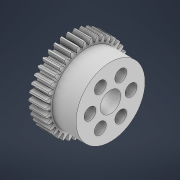
# Autodesk Inventor part: GearWheel
Saved by Autodesk Inventor 2022 (Build 260153000, 153)
## iProperties
Created: 2022-03-28
Part Number: GearWheel
Material: 一般
Document SubType Name: Modeling
Designer: neko2
Density: 1 g/cm^3
Appearance: 既定
Author: neko2
Autodesk Inventor part; units mm, degrees
(part 1 of 4)
ref_plane "YZ Plane" through (0, 0, 0) normal (1, 0, 0) x (0, 1, 0)
ref_plane "XZ Plane" through (0, 0, 0) normal (0, 1, 0) x (-1, 0, 0)
ref_plane "XY Plane" through (0, 0, 0) normal (0, 0, 1) x (1, 0, 0)
sketch "スケッチ1" plane through (0, 0, 0) normal (1, 0, 0) x (0, 1, 0)
  arc A0 (-4.4856, 2.8027) -> (-4.6292, 2.5586) centre (0, 0) ccw
  line L0 (-4.6292, 2.5586) -> (-4.6881, 2.5906)
  spline S0 degree 5 poles (-4.6881, 2.5906) (-4.6897, 2.5915) (-4.693, 2.5932) (-4.698, 2.5957) (-4.7047, 2.5989) (-4.7132, 2.6026) (-4.7219, 2.6061) (-4.7306, 2.6094) (-4.7393, 2.6127) (-4.7481, 2.6159) (-4.7569, 2.6191) (-4.7657, 2.6222) (-4.7746, 2.6252) (-4.7836, 2.6281) (-4.7926, 2.631) (-4.8016, 2.6337) (-4.8107, 2.6364) (-4.8198, 2.639) (-4.8289, 2.6415) (-4.8381, 2.644) (-4.8472, 2.6464) (-4.8565, 2.6488) (-4.8657, 2.6511) (-4.875, 2.6533) (-4.8843, 2.6555) (-4.8936, 2.6576) (-4.903, 2.6597) (-4.9124, 2.6617) (-4.9218, 2.6636) (-4.9313, 2.6656) (-4.9407, 2.6674) (-4.9502, 2.6692) (-4.9597, 2.671) (-4.9693, 2.6727) (-4.9788, 2.6743) (-4.9884, 2.6759) (-4.998, 2.6775) (-5.0076, 2.679) (-5.0173, 2.6804) (-5.027, 2.6818) (-5.0367, 2.6832) (-5.0464, 2.6845) (-5.0561, 2.6858) (-5.0658, 2.687) (-5.0756, 2.6882) (-5.0854, 2.6893) (-5.0952, 2.6904) (-5.105, 2.6915) (-5.1149, 2.6925) (-5.1248, 2.6934) (-5.1346, 2.6943) (-5.1445, 2.6952) (-5.1544, 2.696) (-5.1644, 2.6968) (-5.1743, 2.6976) (-5.1843, 2.6983) (-5.1943, 2.6989) (-5.2043, 2.6995) (-5.2143, 2.7001) (-5.2243, 2.7007) (-5.2344, 2.7012) (-5.2445, 2.7016) (-5.2545, 2.702) (-5.2646, 2.7024) (-5.2747, 2.7027) (-5.2849, 2.703) (-5.295, 2.7033) (-5.3052, 2.7035) (-5.3194, 2.7037) (-5.3316, 2.7039) (-5.3418, 2.704) (-5.35, 2.704) (-5.3562, 2.704) knots 0 0 0 0 0 0 0.014286 0.028571 0.042857 0.057143 0.071429 0.085714 0.1 0.114286 0.128571 0.142857 0.157143 0.171429 0.185714 0.2 0.214286 0.228571 0.242857 0.257143 0.271429 0.285714 0.3 0.314286 0.328571 0.342857 0.357143 0.371429 0.385714 0.4 0.414286 0.428571 0.442857 0.457143 0.471429 0.485714 0.5 0.514286 0.528571 0.542857 0.557143 0.571429 0.585714 0.6 0.614286 0.628571 0.642857 0.657143 0.671429 0.685714 0.7 0.714286 0.728571 0.742857 0.757143 0.771429 0.785714 0.8 0.814286 0.828571 0.842857 0.857143 0.871429 0.885714 0.9 0.914286 0.928571 0.942857 0.957143 1 1 1 1 1 1
  arc A1 (-5.3562, 2.704) -> (-5.4524, 2.5042) centre (0, 0) ccw
  spline S1 degree 5 poles (-4.9475, 2.0523) (-4.9492, 2.0531) (-4.9526, 2.0545) (-4.9576, 2.0569) (-4.9643, 2.0602) (-4.9725, 2.0645) (-4.9806, 2.0691) (-4.9886, 2.0738) (-4.9966, 2.0786) (-5.0046, 2.0835) (-5.0126, 2.0884) (-5.0206, 2.0934) (-5.0285, 2.0984) (-5.0363, 2.1036) (-5.0441, 2.1089) (-5.0519, 2.1142) (-5.0596, 2.1196) (-5.0673, 2.1252) (-5.075, 2.1307) (-5.0827, 2.1363) (-5.0903, 2.142) (-5.0979, 2.1478) (-5.1054, 2.1536) (-5.113, 2.1594) (-5.1205, 2.1653) (-5.128, 2.1713) (-5.1354, 2.1774) (-5.1428, 2.1835) (-5.1502, 2.1896) (-5.1576, 2.1958) (-5.165, 2.2021) (-5.1723, 2.2083) (-5.1796, 2.2147) (-5.1869, 2.2211) (-5.1941, 2.2275) (-5.2013, 2.234) (-5.2085, 2.2406) (-5.2157, 2.2472) (-5.2229, 2.2538) (-5.23, 2.2605) (-5.2371, 2.2672) (-5.2442, 2.274) (-5.2512, 2.2808) (-5.2583, 2.2877) (-5.2653, 2.2946) (-5.2723, 2.3016) (-5.2792, 2.3085) (-5.2862, 2.3156) (-5.2931, 2.3227) (-5.3, 2.3298) (-5.3068, 2.3369) (-5.3137, 2.3441) (-5.3205, 2.3514) (-5.3273, 2.3586) (-5.3341, 2.366) (-5.3409, 2.3733) (-5.3476, 2.3807) (-5.3543, 2.3882) (-5.361, 2.3956) (-5.3677, 2.4031) (-5.3743, 2.4107) (-5.381, 2.4183) (-5.3876, 2.4259) (-5.3942, 2.4336) (-5.4007, 2.4413) (-5.4073, 2.449) (-5.4138, 2.4568) (-5.4203, 2.4646) (-5.4294, 2.4756) (-5.4371, 2.4851) (-5.4435, 2.493) (-5.4486, 2.4994) (-5.4524, 2.5042) knots 0 0 0 0 0 0 0.014286 0.028571 0.042857 0.057143 0.071429 0.085714 0.1 0.114286 0.128571 0.142857 0.157143 0.171429 0.185714 0.2 0.214286 0.228571 0.242857 0.257143 0.271429 0.285714 0.3 0.314286 0.328571 0.342857 0.357143 0.371429 0.385714 0.4 0.414286 0.428571 0.442857 0.457143 0.471429 0.485714 0.5 0.514286 0.528571 0.542857 0.557143 0.571429 0.585714 0.6 0.614286 0.628571 0.642857 0.657143 0.671429 0.685714 0.7 0.714286 0.728571 0.742857 0.757143 0.771429 0.785714 0.8 0.814286 0.828571 0.842857 0.857143 0.871429 0.885714 0.9 0.914286 0.928571 0.942857 0.957143 1 1 1 1 1 1
  line L1 (-4.8857, 2.0262) -> (-4.9475, 2.0523)
  arc A2 (-4.8857, 2.0262) -> (-4.9872, 1.7617) centre (0, 0) ccw
  line L2 (-4.9872, 1.7617) -> (-5.0506, 1.7836)
  spline S2 degree 5 poles (-5.0506, 1.7836) (-5.0523, 1.7842) (-5.0558, 1.7854) (-5.0612, 1.7871) (-5.0683, 1.7891) (-5.0773, 1.7913) (-5.0864, 1.7933) (-5.0955, 1.7952) (-5.1047, 1.797) (-5.1139, 1.7987) (-5.1231, 1.8004) (-5.1323, 1.802) (-5.1416, 1.8035) (-5.1509, 1.805) (-5.1602, 1.8063) (-5.1696, 1.8075) (-5.179, 1.8086) (-5.1884, 1.8097) (-5.1978, 1.8107) (-5.2073, 1.8116) (-5.2167, 1.8125) (-5.2262, 1.8133) (-5.2357, 1.814) (-5.2452, 1.8147) (-5.2548, 1.8154) (-5.2643, 1.8159) (-5.2739, 1.8164) (-5.2835, 1.8168) (-5.2931, 1.8172) (-5.3027, 1.8175) (-5.3124, 1.8178) (-5.322, 1.818) (-5.3317, 1.8182) (-5.3414, 1.8183) (-5.3511, 1.8183) (-5.3608, 1.8183) (-5.3705, 1.8183) (-5.3803, 1.8182) (-5.39, 1.818) (-5.3998, 1.8178) (-5.4096, 1.8176) (-5.4194, 1.8173) (-5.4292, 1.8169) (-5.439, 1.8165) (-5.4489, 1.8161) (-5.4587, 1.8156) (-5.4685, 1.8151) (-5.4784, 1.8145) (-5.4883, 1.8138) (-5.4982, 1.8132) (-5.5081, 1.8124) (-5.518, 1.8117) (-5.5279, 1.8109) (-5.5378, 1.81) (-5.5478, 1.8091) (-5.5577, 1.8082) (-5.5677, 1.8072) (-5.5776, 1.8061) (-5.5876, 1.805) (-5.5976, 1.8039) (-5.6076, 1.8028) (-5.6176, 1.8016) (-5.6276, 1.8003) (-5.6376, 1.799) (-5.6477, 1.7977) (-5.6577, 1.7963) (-5.6677, 1.7949) (-5.6778, 1.7934) (-5.6919, 1.7913) (-5.704, 1.7895) (-5.714, 1.7878) (-5.7221, 1.7865) (-5.7282, 1.7855) knots 0 0 0 0 0 0 0.014286 0.028571 0.042857 0.057143 0.071429 0.085714 0.1 0.114286 0.128571 0.142857 0.157143 0.171429 0.185714 0.2 0.214286 0.228571 0.242857 0.257143 0.271429 0.285714 0.3 0.314286 0.328571 0.342857 0.357143 0.371429 0.385714 0.4 0.414286 0.428571 0.442857 0.457143 0.471429 0.485714 0.5 0.514286 0.528571 0.542857 0.557143 0.571429 0.585714 0.6 0.614286 0.628571 0.642857 0.657143 0.671429 0.685714 0.7 0.714286 0.728571 0.742857 0.757143 0.771429 0.785714 0.8 0.814286 0.828571 0.842857 0.857143 0.871429 0.885714 0.9 0.914286 0.928571 0.942857 0.957143 1 1 1 1 1 1
  arc A3 (-5.7282, 1.7855) -> (-5.7902, 1.5726) centre (0, 0) ccw
  spline S3 degree 5 poles (-5.2178, 1.21) (-5.2196, 1.2105) (-5.2232, 1.2114) (-5.2286, 1.2128) (-5.2357, 1.215) (-5.2445, 1.2179) (-5.2532, 1.2211) (-5.2619, 1.2244) (-5.2706, 1.2278) (-5.2793, 1.2313) (-5.288, 1.2348) (-5.2966, 1.2385) (-5.3053, 1.2422) (-5.3139, 1.246) (-5.3225, 1.2499) (-5.331, 1.2539) (-5.3395, 1.2579) (-5.348, 1.2621) (-5.3565, 1.2663) (-5.365, 1.2706) (-5.3734, 1.275) (-5.3819, 1.2794) (-5.3903, 1.2839) (-5.3987, 1.2884) (-5.4071, 1.293) (-5.4154, 1.2977) (-5.4238, 1.3024) (-5.4321, 1.3072) (-5.4404, 1.312) (-5.4487, 1.3169) (-5.457, 1.3219) (-5.4652, 1.3269) (-5.4735, 1.332) (-5.4817, 1.3371) (-5.4899, 1.3422) (-5.4981, 1.3475) (-5.5063, 1.3527) (-5.5144, 1.3581) (-5.5226, 1.3634) (-5.5307, 1.3689) (-5.5388, 1.3743) (-5.5469, 1.3798) (-5.555, 1.3854) (-5.5631, 1.391) (-5.5711, 1.3967) (-5.5792, 1.4024) (-5.5872, 1.4081) (-5.5952, 1.4139) (-5.6032, 1.4198) (-5.6112, 1.4256) (-5.6191, 1.4316) (-5.6271, 1.4376) (-5.635, 1.4436) (-5.6429, 1.4496) (-5.6508, 1.4557) (-5.6587, 1.4619) (-5.6665, 1.4681) (-5.6744, 1.4743) (-5.6822, 1.4806) (-5.69, 1.4869) (-5.6978, 1.4932) (-5.7056, 1.4996) (-5.7134, 1.5061) (-5.7212, 1.5125) (-5.7289, 1.519) (-5.7366, 1.5256) (-5.7443, 1.5322) (-5.752, 1.5388) (-5.7628, 1.5482) (-5.772, 1.5562) (-5.7796, 1.563) (-5.7857, 1.5685) (-5.7902, 1.5726) knots 0 0 0 0 0 0 0.014286 0.028571 0.042857 0.057143 0.071429 0.085714 0.1 0.114286 0.128571 0.142857 0.157143 0.171429 0.185714 0.2 0.214286 0.228571 0.242857 0.257143 0.271429 0.285714 0.3 0.314286 0.328571 0.342857 0.357143 0.371429 0.385714 0.4 0.414286 0.428571 0.442857 0.457143 0.471429 0.485714 0.5 0.514286 0.528571 0.542857 0.557143 0.571429 0.585714 0.6 0.614286 0.628571 0.642857 0.657143 0.671429 0.685714 0.7 0.714286 0.728571 0.742857 0.757143 0.771429 0.785714 0.8 0.814286 0.828571 0.842857 0.857143 0.871429 0.885714 0.9 0.914286 0.928571 0.942857 0.957143 1 1 1 1 1 1
  line L3 (-5.1526, 1.1944) -> (-5.2178, 1.21)
  arc A4 (-5.1526, 1.1944) -> (-5.2091, 0.9169) centre (0, 0) ccw
  line L4 (-5.2091, 0.9169) -> (-5.2752, 0.928)
  spline S4 degree 5 poles (-5.2752, 0.928) (-5.2771, 0.9283) (-5.2808, 0.9289) (-5.2863, 0.9296) (-5.2937, 0.9305) (-5.3029, 0.9312) (-5.3122, 0.9317) (-5.3215, 0.932) (-5.3308, 0.9323) (-5.3402, 0.9325) (-5.3496, 0.9326) (-5.3589, 0.9327) (-5.3683, 0.9327) (-5.3777, 0.9325) (-5.3872, 0.9323) (-5.3966, 0.9319) (-5.406, 0.9315) (-5.4155, 0.931) (-5.4249, 0.9304) (-5.4344, 0.9298) (-5.4439, 0.9291) (-5.4534, 0.9284) (-5.4629, 0.9275) (-5.4724, 0.9266) (-5.4819, 0.9257) (-5.4914, 0.9247) (-5.501, 0.9236) (-5.5105, 0.9224) (-5.52, 0.9212) (-5.5296, 0.9199) (-5.5391, 0.9186) (-5.5487, 0.9173) (-5.5583, 0.9158) (-5.5678, 0.9143) (-5.5774, 0.9128) (-5.587, 0.9112) (-5.5966, 0.9095) (-5.6062, 0.9078) (-5.6158, 0.9061) (-5.6254, 0.9043) (-5.635, 0.9024) (-5.6446, 0.9005) (-5.6542, 0.8985) (-5.6638, 0.8965) (-5.6735, 0.8945) (-5.6831, 0.8924) (-5.6927, 0.8902) (-5.7023, 0.888) (-5.712, 0.8858) (-5.7216, 0.8835) (-5.7313, 0.8811) (-5.7409, 0.8787) (-5.7506, 0.8763) (-5.7602, 0.8738) (-5.7699, 0.8713) (-5.7795, 0.8687) (-5.7892, 0.8661) (-5.7988, 0.8634) (-5.8085, 0.8607) (-5.8182, 0.858) (-5.8278, 0.8552) (-5.8375, 0.8524) (-5.8472, 0.8495) (-5.8568, 0.8466) (-5.8665, 0.8436) (-5.8762, 0.8406) (-5.8859, 0.8375) (-5.8955, 0.8344) (-5.9091, 0.83) (-5.9207, 0.8262) (-5.9304, 0.823) (-5.9381, 0.8203) (-5.9439, 0.8183) knots 0 0 0 0 0 0 0.014286 0.028571 0.042857 0.057143 0.071429 0.085714 0.1 0.114286 0.128571 0.142857 0.157143 0.171429 0.185714 0.2 0.214286 0.228571 0.242857 0.257143 0.271429 0.285714 0.3 0.314286 0.328571 0.342857 0.357143 0.371429 0.385714 0.4 0.414286 0.428571 0.442857 0.457143 0.471429 0.485714 0.5 0.514286 0.528571 0.542857 0.557143 0.571429 0.585714 0.6 0.614286 0.628571 0.642857 0.657143 0.671429 0.685714 0.7 0.714286 0.728571 0.742857 0.757143 0.771429 0.785714 0.8 0.814286 0.828571 0.842857 0.857143 0.871429 0.885714 0.9 0.914286 0.928571 0.942857 0.957143 1 1 1 1 1 1
  arc A5 (-5.9439, 0.8183) -> (-5.9701, 0.5981) centre (0, 0) ccw
  spline S5 degree 5 poles (-5.3458, 0.3347) (-5.3476, 0.3348) (-5.3513, 0.3351) (-5.3569, 0.3357) (-5.3643, 0.3366) (-5.3734, 0.3381) (-5.3826, 0.3398) (-5.3917, 0.3416) (-5.4008, 0.3436) (-5.41, 0.3456) (-5.4191, 0.3476) (-5.4282, 0.3498) (-5.4374, 0.352) (-5.4465, 0.3543) (-5.4556, 0.3568) (-5.4647, 0.3593) (-5.4737, 0.3619) (-5.4828, 0.3646) (-5.4919, 0.3674) (-5.5009, 0.3702) (-5.51, 0.3731) (-5.519, 0.3761) (-5.5281, 0.3791) (-5.5371, 0.3822) (-5.5461, 0.3854) (-5.5551, 0.3886) (-5.5642, 0.3919) (-5.5732, 0.3953) (-5.5822, 0.3987) (-5.5911, 0.4022) (-5.6001, 0.4057) (-5.6091, 0.4093) (-5.6181, 0.4129) (-5.627, 0.4166) (-5.636, 0.4203) (-5.6449, 0.4241) (-5.6538, 0.428) (-5.6628, 0.4319) (-5.6717, 0.4358) (-5.6806, 0.4399) (-5.6895, 0.4439) (-5.6984, 0.448) (-5.7073, 0.4522) (-5.7162, 0.4564) (-5.725, 0.4606) (-5.7339, 0.4649) (-5.7428, 0.4693) (-5.7516, 0.4737) (-5.7604, 0.4781) (-5.7693, 0.4826) (-5.7781, 0.4872) (-5.7869, 0.4918) (-5.7957, 0.4964) (-5.8045, 0.5011) (-5.8133, 0.5058) (-5.8221, 0.5106) (-5.8309, 0.5154) (-5.8397, 0.5202) (-5.8484, 0.5251) (-5.8572, 0.53) (-5.8659, 0.535) (-5.8746, 0.5401) (-5.8834, 0.5451) (-5.8921, 0.5502) (-5.9008, 0.5554) (-5.9095, 0.5606) (-5.9182, 0.5658) (-5.9269, 0.5711) (-5.939, 0.5785) (-5.9494, 0.585) (-5.958, 0.5904) (-5.9649, 0.5948) (-5.9701, 0.5981) knots 0 0 0 0 0 0 0.014286 0.028571 0.042857 0.057143 0.071429 0.085714 0.1 0.114286 0.128571 0.142857 0.157143 0.171429 0.185714 0.2 0.214286 0.228571 0.242857 0.257143 0.271429 0.285714 0.3 0.314286 0.328571 0.342857 0.357143 0.371429 0.385714 0.4 0.414286 0.428571 0.442857 0.457143 0.471429 0.485714 0.5 0.514286 0.528571 0.542857 0.557143 0.571429 0.585714 0.6 0.614286 0.628571 0.642857 0.657143 0.671429 0.685714 0.7 0.714286 0.728571 0.742857 0.757143 0.771429 0.785714 0.8 0.814286 0.828571 0.842857 0.857143 0.871429 0.885714 0.9 0.914286 0.928571 0.942857 0.957143 1 1 1 1 1 1
  line L5 (-5.2789, 0.33) -> (-5.3458, 0.3347)
  arc A6 (-5.2789, 0.33) -> (-5.289, 0.047) centre (0, 0) ccw
  line L6 (-5.289, 0.047) -> (-5.356, 0.0471)
  spline S6 degree 5 poles (-5.356, 0.0471) (-5.3579, 0.0471) (-5.3616, 0.047) (-5.3672, 0.0469) (-5.3746, 0.0465) (-5.3839, 0.0456) (-5.3931, 0.0446) (-5.4023, 0.0434) (-5.4116, 0.0421) (-5.4208, 0.0408) (-5.4301, 0.0394) (-5.4394, 0.0379) (-5.4486, 0.0363) (-5.4579, 0.0347) (-5.4671, 0.0329) (-5.4764, 0.031) (-5.4856, 0.029) (-5.4949, 0.027) (-5.5041, 0.0248) (-5.5133, 0.0227) (-5.5226, 0.0204) (-5.5318, 0.0181) (-5.541, 0.0157) (-5.5503, 0.0133) (-5.5595, 0.0108) (-5.5687, 0.0082) (-5.5779, 0.0055) (-5.5872, 0.0028) (-5.5964, 0.0001) (-5.6056, -0.0027) (-5.6148, -0.0056) (-5.624, -0.0085) (-5.6332, -0.0115) (-5.6424, -0.0146) (-5.6516, -0.0177) (-5.6608, -0.0208) (-5.67, -0.024) (-5.6791, -0.0273) (-5.6883, -0.0306) (-5.6975, -0.034) (-5.7067, -0.0374) (-5.7158, -0.0409) (-5.725, -0.0444) (-5.7342, -0.0479) (-5.7433, -0.0515) (-5.7525, -0.0552) (-5.7616, -0.0589) (-5.7707, -0.0627) (-5.7799, -0.0665) (-5.789, -0.0703) (-5.7981, -0.0742) (-5.8073, -0.0782) (-5.8164, -0.0822) (-5.8255, -0.0862) (-5.8346, -0.0903) (-5.8437, -0.0944) (-5.8528, -0.0986) (-5.8619, -0.1028) (-5.871, -0.1071) (-5.88, -0.1114) (-5.8891, -0.1157) (-5.8982, -0.1201) (-5.9073, -0.1245) (-5.9163, -0.129) (-5.9254, -0.1335) (-5.9344, -0.1381) (-5.9434, -0.1427) (-5.9525, -0.1473) (-5.9651, -0.1539) (-5.9759, -0.1596) (-5.985, -0.1644) (-5.9922, -0.1683) (-5.9976, -0.1712) knots 0 0 0 0 0 0 0.014286 0.028571 0.042857 0.057143 0.071429 0.085714 0.1 0.114286 0.128571 0.142857 0.157143 0.171429 0.185714 0.2 0.214286 0.228571 0.242857 0.257143 0.271429 0.285714 0.3 0.314286 0.328571 0.342857 0.357143 0.371429 0.385714 0.4 0.414286 0.428571 0.442857 0.457143 0.471429 0.485714 0.5 0.514286 0.528571 0.542857 0.557143 0.571429 0.585714 0.6 0.614286 0.628571 0.642857 0.657143 0.671429 0.685714 0.7 0.714286 0.728571 0.742857 0.757143 0.771429 0.785714 0.8 0.814286 0.828571 0.842857 0.857143 0.871429 0.885714 0.9 0.914286 0.928571 0.942857 0.957143 1 1 1 1 1 1
  arc A7 (-5.9976, -0.1712) -> (-5.9871, -0.3927) centre (0, 0) ccw
  spline S7 degree 5 poles (-5.328, -0.5498) (-5.3298, -0.5499) (-5.3335, -0.5502) (-5.3391, -0.5506) (-5.3465, -0.5509) (-5.3558, -0.5509) (-5.3651, -0.5508) (-5.3744, -0.5505) (-5.3837, -0.5501) (-5.3931, -0.5496) (-5.4024, -0.5491) (-5.4118, -0.5485) (-5.4211, -0.5478) (-5.4305, -0.547) (-5.4399, -0.5461) (-5.4493, -0.545) (-5.4587, -0.5439) (-5.4681, -0.5428) (-5.4775, -0.5415) (-5.4869, -0.5402) (-5.4963, -0.5389) (-5.5057, -0.5374) (-5.5151, -0.5359) (-5.5245, -0.5344) (-5.5339, -0.5327) (-5.5434, -0.531) (-5.5528, -0.5293) (-5.5622, -0.5274) (-5.5716, -0.5255) (-5.5811, -0.5236) (-5.5905, -0.5216) (-5.5999, -0.5196) (-5.6094, -0.5174) (-5.6188, -0.5153) (-5.6283, -0.5131) (-5.6377, -0.5108) (-5.6472, -0.5084) (-5.6566, -0.5061) (-5.6661, -0.5036) (-5.6755, -0.5011) (-5.685, -0.4986) (-5.6944, -0.496) (-5.7039, -0.4934) (-5.7133, -0.4907) (-5.7228, -0.4879) (-5.7322, -0.4852) (-5.7417, -0.4823) (-5.7511, -0.4794) (-5.7606, -0.4765) (-5.77, -0.4735) (-5.7795, -0.4705) (-5.7889, -0.4674) (-5.7984, -0.4643) (-5.8078, -0.4612) (-5.8173, -0.458) (-5.8267, -0.4547) (-5.8362, -0.4514) (-5.8456, -0.4481) (-5.8551, -0.4447) (-5.8645, -0.4412) (-5.874, -0.4378) (-5.8834, -0.4342) (-5.8928, -0.4307) (-5.9023, -0.4271) (-5.9117, -0.4234) (-5.9212, -0.4197) (-5.9306, -0.416) (-5.94, -0.4122) (-5.9532, -0.4069) (-5.9645, -0.4022) (-5.9739, -0.3983) (-5.9815, -0.3951) (-5.9871, -0.3927) knots 0 0 0 0 0 0 0.014286 0.028571 0.042857 0.057143 0.071429 0.085714 0.1 0.114286 0.128571 0.142857 0.157143 0.171429 0.185714 0.2 0.214286 0.228571 0.242857 0.257143 0.271429 0.285714 0.3 0.314286 0.328571 0.342857 0.357143 0.371429 0.385714 0.4 0.414286 0.428571 0.442857 0.457143 0.471429 0.485714 0.5 0.514286 0.528571 0.542857 0.557143 0.571429 0.585714 0.6 0.614286 0.628571 0.642857 0.657143 0.671429 0.685714 0.7 0.714286 0.728571 0.742857 0.757143 0.771429 0.785714 0.8 0.814286 0.828571 0.842857 0.857143 0.871429 0.885714 0.9 0.914286 0.928571 0.942857 0.957143 1 1 1 1 1 1
  line L7 (-5.2612, -0.5434) -> (-5.328, -0.5498)
  arc A8 (-5.2612, -0.5434) -> (-5.2246, -0.8242) centre (0, 0) ccw
  line L8 (-5.2246, -0.8242) -> (-5.2907, -0.8352)
  spline S8 degree 5 poles (-5.2907, -0.8352) (-5.2926, -0.8355) (-5.2962, -0.8361) (-5.3017, -0.8372) (-5.309, -0.8388) (-5.3179, -0.8411) (-5.3269, -0.8437) (-5.3358, -0.8464) (-5.3447, -0.8492) (-5.3536, -0.852) (-5.3625, -0.8549) (-5.3714, -0.8579) (-5.3803, -0.861) (-5.3892, -0.8642) (-5.398, -0.8674) (-5.4068, -0.8708) (-5.4156, -0.8743) (-5.4244, -0.8778) (-5.4331, -0.8814) (-5.4419, -0.8851) (-5.4506, -0.8889) (-5.4593, -0.8926) (-5.4681, -0.8965) (-5.4768, -0.9004) (-5.4854, -0.9044) (-5.4941, -0.9085) (-5.5028, -0.9126) (-5.5114, -0.9168) (-5.5201, -0.9211) (-5.5287, -0.9253) (-5.5373, -0.9297) (-5.5459, -0.9341) (-5.5545, -0.9386) (-5.563, -0.9431) (-5.5716, -0.9477) (-5.5801, -0.9523) (-5.5887, -0.957) (-5.5972, -0.9617) (-5.6057, -0.9665) (-5.6142, -0.9713) (-5.6227, -0.9762) (-5.6312, -0.9811) (-5.6396, -0.9861) (-5.6481, -0.9911) (-5.6565, -0.9962) (-5.6649, -1.0013) (-5.6733, -1.0064) (-5.6817, -1.0116) (-5.6901, -1.0169) (-5.6985, -1.0222) (-5.7068, -1.0276) (-5.7152, -1.0329) (-5.7235, -1.0384) (-5.7318, -1.0439) (-5.7402, -1.0494) (-5.7485, -1.055) (-5.7567, -1.0606) (-5.765, -1.0662) (-5.7733, -1.0719) (-5.7815, -1.0777) (-5.7898, -1.0834) (-5.798, -1.0893) (-5.8062, -1.0951) (-5.8144, -1.101) (-5.8226, -1.107) (-5.8307, -1.113) (-5.8389, -1.119) (-5.847, -1.1251) (-5.8584, -1.1336) (-5.8682, -1.141) (-5.8763, -1.1472) (-5.8827, -1.1522) (-5.8876, -1.156) knots 0 0 0 0 0 0 0.014286 0.028571 0.042857 0.057143 0.071429 0.085714 0.1 0.114286 0.128571 0.142857 0.157143 0.171429 0.185714 0.2 0.214286 0.228571 0.242857 0.257143 0.271429 0.285714 0.3 0.314286 0.328571 0.342857 0.357143 0.371429 0.385714 0.4 0.414286 0.428571 0.442857 0.457143 0.471429 0.485714 0.5 0.514286 0.528571 0.542857 0.557143 0.571429 0.585714 0.6 0.614286 0.628571 0.642857 0.657143 0.671429 0.685714 0.7 0.714286 0.728571 0.742857 0.757143 0.771429 0.785714 0.8 0.814286 0.828571 0.842857 0.857143 0.871429 0.885714 0.9 0.914286 0.928571 0.942857 0.957143 1 1 1 1 1 1
  arc A9 (-5.8876, -1.156) -> (-5.8408, -1.3728) centre (0, 0) ccw
  spline S9 degree 5 poles (-5.1648, -1.4192) (-5.1666, -1.4197) (-5.1702, -1.4206) (-5.1756, -1.4219) (-5.1829, -1.4234) (-5.1921, -1.425) (-5.2013, -1.4263) (-5.2105, -1.4276) (-5.2198, -1.4287) (-5.2291, -1.4298) (-5.2384, -1.4308) (-5.2477, -1.4317) (-5.257, -1.4326) (-5.2664, -1.4333) (-5.2758, -1.434) (-5.2852, -1.4345) (-5.2947, -1.435) (-5.3041, -1.4354) (-5.3136, -1.4357) (-5.3231, -1.436) (-5.3326, -1.4362) (-5.3421, -1.4363) (-5.3517, -1.4364) (-5.3612, -1.4364) (-5.3708, -1.4363) (-5.3803, -1.4362) (-5.3899, -1.436) (-5.3995, -1.4357) (-5.4091, -1.4354) (-5.4188, -1.4351) (-5.4284, -1.4347) (-5.4381, -1.4342) (-5.4477, -1.4337) (-5.4574, -1.4331) (-5.4671, -1.4324) (-5.4768, -1.4317) (-5.4865, -1.431) (-5.4962, -1.4302) (-5.5059, -1.4294) (-5.5156, -1.4285) (-5.5254, -1.4275) (-5.5351, -1.4265) (-5.5449, -1.4255) (-5.5546, -1.4244) (-5.5644, -1.4232) (-5.5742, -1.422) (-5.584, -1.4208) (-5.5938, -1.4195) (-5.6036, -1.4182) (-5.6134, -1.4168) (-5.6232, -1.4154) (-5.633, -1.4139) (-5.6429, -1.4124) (-5.6527, -1.4108) (-5.6626, -1.4092) (-5.6724, -1.4075) (-5.6823, -1.4058) (-5.6922, -1.4041) (-5.702, -1.4023) (-5.7119, -1.4005) (-5.7218, -1.3986) (-5.7317, -1.3967) (-5.7416, -1.3947) (-5.7515, -1.3927) (-5.7614, -1.3907) (-5.7713, -1.3886) (-5.7812, -1.3865) (-5.7912, -1.3843) (-5.8051, -1.3812) (-5.817, -1.3785) (-5.8269, -1.3761) (-5.8349, -1.3743) (-5.8408, -1.3728) knots 0 0 0 0 0 0 0.014286 0.028571 0.042857 0.057143 0.071429 0.085714 0.1 0.114286 0.128571 0.142857 0.157143 0.171429 0.185714 0.2 0.214286 0.228571 0.242857 0.257143 0.271429 0.285714 0.3 0.314286 0.328571 0.342857 0.357143 0.371429 0.385714 0.4 0.414286 0.428571 0.442857 0.457143 0.471429 0.485714 0.5 0.514286 0.528571 0.542857 0.557143 0.571429 0.585714 0.6 0.614286 0.628571 0.642857 0.657143 0.671429 0.685714 0.7 0.714286 0.728571 0.742857 0.757143 0.771429 0.785714 0.8 0.814286 0.828571 0.842857 0.857143 0.871429 0.885714 0.9 0.914286 0.928571 0.942857 0.957143 1 1 1 1 1 1
  line L9 (-5.1, -1.4019) -> (-5.1648, -1.4192)
  arc A10 (-5.1, -1.4019) -> (-5.0177, -1.6729) centre (0, 0) ccw
  line L10 (-5.0177, -1.6729) -> (-5.0811, -1.6946)
  spline S10 degree 5 poles (-5.0811, -1.6946) (-5.0829, -1.6952) (-5.0864, -1.6964) (-5.0916, -1.6984) (-5.0985, -1.7012) (-5.107, -1.705) (-5.1154, -1.709) (-5.1237, -1.7131) (-5.1321, -1.7173) (-5.1404, -1.7216) (-5.1487, -1.7259) (-5.157, -1.7303) (-5.1652, -1.7348) (-5.1734, -1.7394) (-5.1816, -1.7441) (-5.1897, -1.7489) (-5.1978, -1.7537) (-5.2059, -1.7587) (-5.2139, -1.7637) (-5.222, -1.7687) (-5.23, -1.7739) (-5.238, -1.7791) (-5.2459, -1.7843) (-5.2539, -1.7896) (-5.2618, -1.795) (-5.2697, -1.8004) (-5.2775, -1.8059) (-5.2854, -1.8115) (-5.2932, -1.8171) (-5.301, -1.8227) (-5.3087, -1.8284) (-5.3165, -1.8342) (-5.3242, -1.84) (-5.3319, -1.8459) (-5.3396, -1.8518) (-5.3473, -1.8578) (-5.3549, -1.8638) (-5.3626, -1.8698) (-5.3702, -1.8759) (-5.3778, -1.8821) (-5.3853, -1.8883) (-5.3929, -1.8946) (-5.4004, -1.9009) (-5.4079, -1.9072) (-5.4154, -1.9136) (-5.4228, -1.92) (-5.4303, -1.9265) (-5.4377, -1.933) (-5.4451, -1.9396) (-5.4525, -1.9462) (-5.4599, -1.9529) (-5.4672, -1.9595) (-5.4745, -1.9663) (-5.4819, -1.9731) (-5.4891, -1.9799) (-5.4964, -1.9867) (-5.5037, -1.9936) (-5.5109, -2.0006) (-5.5181, -2.0075) (-5.5253, -2.0146) (-5.5325, -2.0216) (-5.5396, -2.0287) (-5.5467, -2.0359) (-5.5539, -2.043) (-5.561, -2.0502) (-5.568, -2.0575) (-5.5751, -2.0648) (-5.5821, -2.0721) (-5.5919, -2.0824) (-5.6003, -2.0913) (-5.6073, -2.0988) (-5.6129, -2.1048) (-5.617, -2.1093) knots 0 0 0 0 0 0 0.014286 0.028571 0.042857 0.057143 0.071429 0.085714 0.1 0.114286 0.128571 0.142857 0.157143 0.171429 0.185714 0.2 0.214286 0.228571 0.242857 0.257143 0.271429 0.285714 0.3 0.314286 0.328571 0.342857 0.357143 0.371429 0.385714 0.4 0.414286 0.428571 0.442857 0.457143 0.471429 0.485714 0.5 0.514286 0.528571 0.542857 0.557143 0.571429 0.585714 0.6 0.614286 0.628571 0.642857 0.657143 0.671429 0.685714 0.7 0.714286 0.728571 0.742857 0.757143 0.771429 0.785714 0.8 0.814286 0.828571 0.842857 0.857143 0.871429 0.885714 0.9 0.914286 0.928571 0.942857 0.957143 1 1 1 1 1 1
  arc A11 (-5.617, -2.1093) -> (-5.5352, -2.3155) centre (0, 0) ccw
  spline S11 degree 5 poles (-4.8608, -2.25) (-4.8625, -2.2507) (-4.8659, -2.2522) (-4.871, -2.2544) (-4.8779, -2.2571) (-4.8867, -2.2601) (-4.8956, -2.263) (-4.9045, -2.2657) (-4.9134, -2.2684) (-4.9224, -2.2709) (-4.9314, -2.2735) (-4.9405, -2.2759) (-4.9496, -2.2783) (-4.9587, -2.2806) (-4.9678, -2.2828) (-4.977, -2.2849) (-4.9863, -2.2869) (-4.9955, -2.2888) (-5.0048, -2.2907) (-5.0142, -2.2925) (-5.0235, -2.2943) (-5.0329, -2.296) (-5.0422, -2.2976) (-5.0517, -2.2992) (-5.0611, -2.3007) (-5.0706, -2.3022) (-5.0801, -2.3036) (-5.0896, -2.3049) (-5.0991, -2.3062) (-5.1087, -2.3074) (-5.1182, -2.3086) (-5.1278, -2.3097) (-5.1374, -2.3108) (-5.1471, -2.3118) (-5.1567, -2.3128) (-5.1664, -2.3137) (-5.1761, -2.3145) (-5.1858, -2.3153) (-5.1955, -2.3161) (-5.2053, -2.3168) (-5.215, -2.3175) (-5.2248, -2.3181) (-5.2346, -2.3187) (-5.2444, -2.3192) (-5.2543, -2.3197) (-5.2641, -2.3201) (-5.274, -2.3205) (-5.2838, -2.3209) (-5.2937, -2.3212) (-5.3036, -2.3214) (-5.3136, -2.3216) (-5.3235, -2.3218) (-5.3335, -2.3219) (-5.3434, -2.322) (-5.3534, -2.322) (-5.3634, -2.322) (-5.3734, -2.3219) (-5.3834, -2.3219) (-5.3934, -2.3217) (-5.4035, -2.3215) (-5.4136, -2.3213) (-5.4236, -2.3211) (-5.4337, -2.3208) (-5.4438, -2.3204) (-5.4539, -2.32) (-5.464, -2.3196) (-5.4742, -2.3191) (-5.4843, -2.3186) (-5.4985, -2.3178) (-5.5107, -2.3171) (-5.5209, -2.3165) (-5.5291, -2.3159) (-5.5352, -2.3155) knots 0 0 0 0 0 0 0.014286 0.028571 0.042857 0.057143 0.071429 0.085714 0.1 0.114286 0.128571 0.142857 0.157143 0.171429 0.185714 0.2 0.214286 0.228571 0.242857 0.257143 0.271429 0.285714 0.3 0.314286 0.328571 0.342857 0.357143 0.371429 0.385714 0.4 0.414286 0.428571 0.442857 0.457143 0.471429 0.485714 0.5 0.514286 0.528571 0.542857 0.557143 0.571429 0.585714 0.6 0.614286 0.628571 0.642857 0.657143 0.671429 0.685714 0.7 0.714286 0.728571 0.742857 0.757143 0.771429 0.785714 0.8 0.814286 0.828571 0.842857 0.857143 0.871429 0.885714 0.9 0.914286 0.928571 0.942857 0.957143 1 1 1 1 1 1
  line L11 (-4.7997, -2.2222) -> (-4.8608, -2.25)
  arc A12 (-4.7997, -2.2222) -> (-4.6739, -2.476) centre (0, 0) ccw
  line L12 (-4.6739, -2.476) -> (-4.7329, -2.5078)
  spline S12 degree 5 poles (-4.7329, -2.5078) (-4.7345, -2.5087) (-4.7378, -2.5105) (-4.7426, -2.5133) (-4.7489, -2.5172) (-4.7567, -2.5223) (-4.7643, -2.5276) (-4.7719, -2.533) (-4.7794, -2.5386) (-4.7869, -2.5442) (-4.7944, -2.5498) (-4.8018, -2.5555) (-4.8092, -2.5613) (-4.8166, -2.5672) (-4.8238, -2.5732) (-4.8311, -2.5792) (-4.8383, -2.5854) (-4.8454, -2.5916) (-4.8525, -2.5978) (-4.8596, -2.6041) (-4.8667, -2.6105) (-4.8737, -2.6169) (-4.8807, -2.6234) (-4.8876, -2.63) (-4.8946, -2.6366) (-4.9014, -2.6432) (-4.9083, -2.6499) (-4.9151, -2.6567) (-4.9219, -2.6635) (-4.9287, -2.6704) (-4.9354, -2.6773) (-4.9421, -2.6842) (-4.9488, -2.6912) (-4.9554, -2.6983) (-4.962, -2.7054) (-4.9686, -2.7125) (-4.9751, -2.7197) (-4.9817, -2.727) (-4.9882, -2.7343) (-4.9946, -2.7416) (-5.0011, -2.749) (-5.0075, -2.7564) (-5.0139, -2.7638) (-5.0202, -2.7713) (-5.0266, -2.7788) (-5.0329, -2.7864) (-5.0391, -2.794) (-5.0454, -2.8017) (-5.0516, -2.8094) (-5.0578, -2.8171) (-5.064, -2.8249) (-5.0701, -2.8327) (-5.0762, -2.8405) (-5.0823, -2.8484) (-5.0884, -2.8564) (-5.0944, -2.8643) (-5.1005, -2.8723) (-5.1064, -2.8803) (-5.1124, -2.8884) (-5.1183, -2.8965) (-5.1243, -2.9047) (-5.1301, -2.9128) (-5.136, -2.9211) (-5.1418, -2.9293) (-5.1477, -2.9376) (-5.1534, -2.9459) (-5.1592, -2.9542) (-5.1649, -2.9626) (-5.1729, -2.9744) (-5.1797, -2.9846) (-5.1854, -2.9931) (-5.1899, -2.9999) (-5.1932, -3.0051) knots 0 0 0 0 0 0 0.014286 0.028571 0.042857 0.057143 0.071429 0.085714 0.1 0.114286 0.128571 0.142857 0.157143 0.171429 0.185714 0.2 0.214286 0.228571 0.242857 0.257143 0.271429 0.285714 0.3 0.314286 0.328571 0.342857 0.357143 0.371429 0.385714 0.4 0.414286 0.428571 0.442857 0.457143 0.471429 0.485714 0.5 0.514286 0.528571 0.542857 0.557143 0.571429 0.585714 0.6 0.614286 0.628571 0.642857 0.657143 0.671429 0.685714 0.7 0.714286 0.728571 0.742857 0.757143 0.771429 0.785714 0.8 0.814286 0.828571 0.842857 0.857143 0.871429 0.885714 0.9 0.914286 0.928571 0.942857 0.957143 1 1 1 1 1 1
  arc A13 (-5.1932, -3.0051) -> (-5.0786, -3.1949) centre (0, 0) ccw
  spline S13 degree 5 poles (-4.4241, -3.0193) (-4.4257, -3.0204) (-4.4288, -3.0224) (-4.4335, -3.0254) (-4.4399, -3.0292) (-4.4481, -3.0336) (-4.4563, -3.0379) (-4.4647, -3.0421) (-4.473, -3.0461) (-4.4815, -3.0502) (-4.49, -3.0542) (-4.4985, -3.0581) (-4.507, -3.0619) (-4.5157, -3.0657) (-4.5244, -3.0693) (-4.5331, -3.0729) (-4.5419, -3.0764) (-4.5507, -3.0799) (-4.5595, -3.0832) (-4.5684, -3.0866) (-4.5773, -3.0898) (-4.5863, -3.0931) (-4.5953, -3.0962) (-4.6043, -3.0993) (-4.6134, -3.1024) (-4.6225, -3.1054) (-4.6316, -3.1083) (-4.6408, -3.1112) (-4.65, -3.114) (-4.6592, -3.1168) (-4.6684, -3.1195) (-4.6777, -3.1222) (-4.687, -3.1248) (-4.6964, -3.1274) (-4.7057, -3.13) (-4.7151, -3.1325) (-4.7245, -3.1349) (-4.734, -3.1373) (-4.7435, -3.1397) (-4.753, -3.142) (-4.7625, -3.1442) (-4.772, -3.1465) (-4.7816, -3.1486) (-4.7912, -3.1508) (-4.8008, -3.1529) (-4.8104, -3.1549) (-4.8201, -3.1569) (-4.8298, -3.1589) (-4.8395, -3.1608) (-4.8492, -3.1627) (-4.859, -3.1645) (-4.8687, -3.1663) (-4.8785, -3.1681) (-4.8884, -3.1698) (-4.8982, -3.1715) (-4.9081, -3.1731) (-4.9179, -3.1747) (-4.9278, -3.1763) (-4.9377, -3.1778) (-4.9477, -3.1793) (-4.9576, -3.1807) (-4.9676, -3.1821) (-4.9776, -3.1835) (-4.9876, -3.1848) (-4.9977, -3.1861) (-5.0077, -3.1873) (-5.0178, -3.1885) (-5.0279, -3.1897) (-5.042, -3.1913) (-5.0542, -3.1926) (-5.0644, -3.1936) (-5.0725, -3.1944) (-5.0786, -3.1949) knots 0 0 0 0 0 0 0.014286 0.028571 0.042857 0.057143 0.071429 0.085714 0.1 0.114286 0.128571 0.142857 0.157143 0.171429 0.185714 0.2 0.214286 0.228571 0.242857 0.257143 0.271429 0.285714 0.3 0.314286 0.328571 0.342857 0.357143 0.371429 0.385714 0.4 0.414286 0.428571 0.442857 0.457143 0.471429 0.485714 0.5 0.514286 0.528571 0.542857 0.557143 0.571429 0.585714 0.6 0.614286 0.628571 0.642857 0.657143 0.671429 0.685714 0.7 0.714286 0.728571 0.742857 0.757143 0.771429 0.785714 0.8 0.814286 0.828571 0.842857 0.857143 0.871429 0.885714 0.9 0.914286 0.928571 0.942857 0.957143 1 1 1 1 1 1
  line L13 (-4.3685, -2.9819) -> (-4.4241, -3.0193)
  arc A14 (-4.3685, -2.9819) -> (-4.2026, -3.2115) centre (0, 0) ccw
  line L14 (-4.2026, -3.2115) -> (-4.2556, -3.2526)
  spline S14 degree 5 poles (-4.2556, -3.2526) (-4.257, -3.2538) (-4.26, -3.2561) (-4.2643, -3.2596) (-4.2699, -3.2645) (-4.2767, -3.2708) (-4.2833, -3.2773) (-4.2899, -3.2839) (-4.2964, -3.2906) (-4.3029, -3.2974) (-4.3093, -3.3042) (-4.3157, -3.311) (-4.3221, -3.3179) (-4.3283, -3.325) (-4.3345, -3.332) (-4.3407, -3.3392) (-4.3467, -3.3464) (-4.3528, -3.3537) (-4.3588, -3.3611) (-4.3647, -3.3685) (-4.3706, -3.3759) (-4.3765, -3.3834) (-4.3823, -3.391) (-4.3881, -3.3986) (-4.3938, -3.4062) (-4.3995, -3.4139) (-4.4052, -3.4217) (-4.4108, -3.4295) (-4.4164, -3.4373) (-4.4219, -3.4452) (-4.4274, -3.4531) (-4.4329, -3.4611) (-4.4383, -3.4691) (-4.4437, -3.4771) (-4.449, -3.4852) (-4.4544, -3.4934) (-4.4596, -3.5015) (-4.4649, -3.5097) (-4.4701, -3.518) (-4.4753, -3.5263) (-4.4804, -3.5346) (-4.4855, -3.543) (-4.4906, -3.5514) (-4.4956, -3.5598) (-4.5006, -3.5683) (-4.5056, -3.5768) (-4.5105, -3.5853) (-4.5154, -3.5939) (-4.5203, -3.6025) (-4.5251, -3.6112) (-4.53, -3.6199) (-4.5347, -3.6286) (-4.5395, -3.6373) (-4.5442, -3.6461) (-4.5489, -3.6549) (-4.5535, -3.6638) (-4.5581, -3.6726) (-4.5627, -3.6816) (-4.5673, -3.6905) (-4.5718, -3.6995) (-4.5763, -3.7085) (-4.5807, -3.7175) (-4.5852, -3.7266) (-4.5896, -3.7357) (-4.5939, -3.7448) (-4.5983, -3.7539) (-4.6026, -3.7631) (-4.6069, -3.7723) (-4.6128, -3.7853) (-4.6178, -3.7964) (-4.622, -3.8058) (-4.6253, -3.8132) (-4.6278, -3.8189) knots 0 0 0 0 0 0 0.014286 0.028571 0.042857 0.057143 0.071429 0.085714 0.1 0.114286 0.128571 0.142857 0.157143 0.171429 0.185714 0.2 0.214286 0.228571 0.242857 0.257143 0.271429 0.285714 0.3 0.314286 0.328571 0.342857 0.357143 0.371429 0.385714 0.4 0.414286 0.428571 0.442857 0.457143 0.471429 0.485714 0.5 0.514286 0.528571 0.542857 0.557143 0.571429 0.585714 0.6 0.614286 0.628571 0.642857 0.657143 0.671429 0.685714 0.7 0.714286 0.728571 0.742857 0.757143 0.771429 0.785714 0.8 0.814286 0.828571 0.842857 0.857143 0.871429 0.885714 0.9 0.914286 0.928571 0.942857 0.957143 1 1 1 1 1 1
  arc A15 (-4.6278, -3.8189) -> (-4.4835, -3.9873) centre (0, 0) ccw
  spline S15 degree 5 poles (-3.8668, -3.7063) (-3.8682, -3.7076) (-3.8709, -3.7101) (-3.8751, -3.7138) (-3.8808, -3.7186) (-3.8881, -3.7244) (-3.8955, -3.73) (-3.9031, -3.7354) (-3.9107, -3.7408) (-3.9183, -3.7462) (-3.926, -3.7515) (-3.9338, -3.7568) (-3.9416, -3.762) (-3.9495, -3.7671) (-3.9574, -3.7722) (-3.9655, -3.7771) (-3.9736, -3.782) (-3.9817, -3.7869) (-3.9899, -3.7917) (-3.9981, -3.7964) (-4.0063, -3.8011) (-4.0147, -3.8058) (-4.023, -3.8104) (-4.0314, -3.8149) (-4.0398, -3.8194) (-4.0483, -3.8238) (-4.0568, -3.8282) (-4.0654, -3.8326) (-4.074, -3.8369) (-4.0826, -3.8412) (-4.0913, -3.8454) (-4.1, -3.8496) (-4.1088, -3.8537) (-4.1176, -3.8578) (-4.1264, -3.8618) (-4.1352, -3.8658) (-4.1441, -3.8698) (-4.153, -3.8737) (-4.162, -3.8776) (-4.171, -3.8814) (-4.18, -3.8852) (-4.189, -3.889) (-4.1981, -3.8927) (-4.2072, -3.8964) (-4.2164, -3.9001) (-4.2255, -3.9037) (-4.2347, -3.9072) (-4.244, -3.9108) (-4.2532, -3.9143) (-4.2625, -3.9177) (-4.2718, -3.9211) (-4.2812, -3.9245) (-4.2906, -3.9279) (-4.3, -3.9312) (-4.3094, -3.9344) (-4.3188, -3.9377) (-4.3283, -3.9409) (-4.3378, -3.944) (-4.3474, -3.9472) (-4.3569, -3.9503) (-4.3665, -3.9533) (-4.3761, -3.9563) (-4.3858, -3.9593) (-4.3954, -3.9623) (-4.4051, -3.9652) (-4.4148, -3.9681) (-4.4246, -3.9709) (-4.4343, -3.9737) (-4.448, -3.9776) (-4.4598, -3.9809) (-4.4696, -3.9836) (-4.4775, -3.9857) (-4.4835, -3.9873) knots 0 0 0 0 0 0 0.014286 0.028571 0.042857 0.057143 0.071429 0.085714 0.1 0.114286 0.128571 0.142857 0.157143 0.171429 0.185714 0.2 0.214286 0.228571 0.242857 0.257143 0.271429 0.285714 0.3 0.314286 0.328571 0.342857 0.357143 0.371429 0.385714 0.4 0.414286 0.428571 0.442857 0.457143 0.471429 0.485714 0.5 0.514286 0.528571 0.542857 0.557143 0.571429 0.585714 0.6 0.614286 0.628571 0.642857 0.657143 0.671429 0.685714 0.7 0.714286 0.728571 0.742857 0.757143 0.771429 0.785714 0.8 0.814286 0.828571 0.842857 0.857143 0.871429 0.885714 0.9 0.914286 0.928571 0.942857 0.957143 1 1 1 1 1 1
  line L15 (-3.8181, -3.6603) -> (-3.8668, -3.7063)
  arc A16 (-3.8181, -3.6603) -> (-3.6167, -3.8594) centre (0, 0) ccw
  line L16 (-3.6167, -3.8594) -> (-3.6622, -3.9087)
  spline S16 degree 5 poles (-3.6622, -3.9087) (-3.6634, -3.9101) (-3.6659, -3.9128) (-3.6696, -3.917) (-3.6743, -3.9228) (-3.68, -3.9301) (-3.6855, -3.9376) (-3.6908, -3.9452) (-3.6962, -3.9529) (-3.7015, -3.9606) (-3.7067, -3.9684) (-3.7119, -3.9762) (-3.717, -3.9841) (-3.722, -3.992) (-3.727, -4) (-3.7318, -4.0081) (-3.7367, -4.0163) (-3.7414, -4.0244) (-3.7461, -4.0327) (-3.7508, -4.0409) (-3.7554, -4.0493) (-3.7599, -4.0576) (-3.7644, -4.066) (-3.7689, -4.0745) (-3.7733, -4.083) (-3.7776, -4.0915) (-3.7819, -4.1001) (-3.7862, -4.1087) (-3.7904, -4.1173) (-3.7945, -4.126) (-3.7987, -4.1347) (-3.8027, -4.1435) (-3.8068, -4.1523) (-3.8108, -4.1611) (-3.8147, -4.17) (-3.8186, -4.1789) (-3.8225, -4.1878) (-3.8263, -4.1968) (-3.8301, -4.2058) (-3.8338, -4.2148) (-3.8375, -4.2238) (-3.8412, -4.2329) (-3.8448, -4.2421) (-3.8484, -4.2512) (-3.8519, -4.2604) (-3.8554, -4.2696) (-3.8589, -4.2788) (-3.8623, -4.2881) (-3.8657, -4.2974) (-3.869, -4.3067) (-3.8724, -4.3161) (-3.8756, -4.3255) (-3.8789, -4.3349) (-3.8821, -4.3443) (-3.8852, -4.3538) (-3.8884, -4.3633) (-3.8915, -4.3728) (-3.8945, -4.3823) (-3.8975, -4.3919) (-3.9005, -4.4015) (-3.9035, -4.4111) (-3.9064, -4.4208) (-3.9093, -4.4304) (-3.9121, -4.4401) (-3.9149, -4.4499) (-3.9177, -4.4596) (-3.9204, -4.4694) (-3.9231, -4.4792) (-3.9269, -4.4929) (-3.93, -4.5047) (-3.9326, -4.5146) (-3.9346, -4.5225) (-3.9361, -4.5285) knots 0 0 0 0 0 0 0.014286 0.028571 0.042857 0.057143 0.071429 0.085714 0.1 0.114286 0.128571 0.142857 0.157143 0.171429 0.185714 0.2 0.214286 0.228571 0.242857 0.257143 0.271429 0.285714 0.3 0.314286 0.328571 0.342857 0.357143 0.371429 0.385714 0.4 0.414286 0.428571 0.442857 0.457143 0.471429 0.485714 0.5 0.514286 0.528571 0.542857 0.557143 0.571429 0.585714 0.6 0.614286 0.628571 0.642857 0.657143 0.671429 0.685714 0.7 0.714286 0.728571 0.742857 0.757143 0.771429 0.785714 0.8 0.814286 0.828571 0.842857 0.857143 0.871429 0.885714 0.9 0.914286 0.928571 0.942857 0.957143 1 1 1 1 1 1
  arc A17 (-3.9361, -4.5285) -> (-3.766, -4.6709) centre (0, 0) ccw
  spline S17 degree 5 poles (-3.2041, -4.2922) (-3.2052, -4.2937) (-3.2075, -4.2967) (-3.211, -4.301) (-3.2158, -4.3067) (-3.222, -4.3135) (-3.2285, -4.3203) (-3.235, -4.3269) (-3.2416, -4.3335) (-3.2483, -4.34) (-3.255, -4.3466) (-3.2618, -4.353) (-3.2686, -4.3595) (-3.2756, -4.3658) (-3.2826, -4.3721) (-3.2897, -4.3783) (-3.2969, -4.3845) (-3.3041, -4.3906) (-3.3114, -4.3967) (-3.3187, -4.4027) (-3.3261, -4.4087) (-3.3335, -4.4146) (-3.341, -4.4206) (-3.3485, -4.4264) (-3.3561, -4.4322) (-3.3637, -4.438) (-3.3714, -4.4438) (-3.3791, -4.4495) (-3.3869, -4.4551) (-3.3947, -4.4608) (-3.4026, -4.4663) (-3.4105, -4.4719) (-3.4184, -4.4774) (-3.4264, -4.4829) (-3.4345, -4.4883) (-3.4425, -4.4937) (-3.4506, -4.4991) (-3.4588, -4.5045) (-3.467, -4.5098) (-3.4752, -4.515) (-3.4835, -4.5203) (-3.4918, -4.5255) (-3.5001, -4.5306) (-3.5085, -4.5358) (-3.5169, -4.5409) (-3.5254, -4.5459) (-3.5339, -4.551) (-3.5424, -4.556) (-3.551, -4.5609) (-3.5595, -4.5659) (-3.5682, -4.5708) (-3.5768, -4.5756) (-3.5855, -4.5805) (-3.5943, -4.5853) (-3.603, -4.5901) (-3.6118, -4.5948) (-3.6206, -4.5995) (-3.6295, -4.6042) (-3.6384, -4.6089) (-3.6473, -4.6135) (-3.6563, -4.6181) (-3.6652, -4.6227) (-3.6743, -4.6272) (-3.6833, -4.6317) (-3.6924, -4.6362) (-3.7015, -4.6406) (-3.7106, -4.645) (-3.7198, -4.6494) (-3.7326, -4.6555) (-3.7437, -4.6607) (-3.753, -4.6649) (-3.7604, -4.6683) (-3.766, -4.6709) knots 0 0 0 0 0 0 0.014286 0.028571 0.042857 0.057143 0.071429 0.085714 0.1 0.114286 0.128571 0.142857 0.157143 0.171429 0.185714 0.2 0.214286 0.228571 0.242857 0.257143 0.271429 0.285714 0.3 0.314286 0.328571 0.342857 0.357143 0.371429 0.385714 0.4 0.414286 0.428571 0.442857 0.457143 0.471429 0.485714 0.5 0.514286 0.528571 0.542857 0.557143 0.571429 0.585714 0.6 0.614286 0.628571 0.642857 0.657143 0.671429 0.685714 0.7 0.714286 0.728571 0.742857 0.757143 0.771429 0.785714 0.8 0.814286 0.828571 0.842857 0.857143 0.871429 0.885714 0.9 0.914286 0.928571 0.942857 0.957143 1 1 1 1 1 1
  line L17 (-3.1636, -4.2388) -> (-3.2041, -4.2922)
  arc A18 (-3.1636, -4.2388) -> (-2.9321, -4.4021) centre (0, 0) ccw
  line L18 (-2.9321, -4.4021) -> (-2.9689, -4.4582)
  spline S18 degree 5 poles (-2.9689, -4.4582) (-2.9699, -4.4597) (-2.9719, -4.4628) (-2.9748, -4.4676) (-2.9785, -4.474) (-2.9829, -4.4822) (-2.9871, -4.4905) (-2.9911, -4.4989) (-2.9951, -4.5074) (-2.9991, -4.5158) (-3.003, -4.5244) (-3.0068, -4.5329) (-3.0105, -4.5415) (-3.0142, -4.5502) (-3.0178, -4.5589) (-3.0212, -4.5677) (-3.0246, -4.5765) (-3.028, -4.5854) (-3.0313, -4.5943) (-3.0345, -4.6032) (-3.0377, -4.6121) (-3.0408, -4.6211) (-3.0438, -4.6302) (-3.0468, -4.6392) (-3.0498, -4.6483) (-3.0527, -4.6575) (-3.0555, -4.6666) (-3.0583, -4.6758) (-3.061, -4.685) (-3.0637, -4.6943) (-3.0663, -4.7036) (-3.0689, -4.7129) (-3.0714, -4.7222) (-3.0739, -4.7316) (-3.0763, -4.741) (-3.0787, -4.7504) (-3.0811, -4.7598) (-3.0833, -4.7693) (-3.0856, -4.7788) (-3.0878, -4.7883) (-3.09, -4.7979) (-3.0921, -4.8074) (-3.0941, -4.817) (-3.0962, -4.8267) (-3.0981, -4.8363) (-3.1001, -4.846) (-3.102, -4.8556) (-3.1038, -4.8653) (-3.1056, -4.8751) (-3.1074, -4.8848) (-3.1091, -4.8946) (-3.1108, -4.9044) (-3.1125, -4.9142) (-3.1141, -4.924) (-3.1156, -4.9339) (-3.1172, -4.9438) (-3.1186, -4.9537) (-3.1201, -4.9636) (-3.1215, -4.9735) (-3.1229, -4.9835) (-3.1242, -4.9935) (-3.1255, -5.0034) (-3.1267, -5.0135) (-3.1279, -5.0235) (-3.1291, -5.0335) (-3.1302, -5.0436) (-3.1313, -5.0537) (-3.1324, -5.0638) (-3.1338, -5.078) (-3.1349, -5.0901) (-3.1358, -5.1003) (-3.1365, -5.1085) (-3.1371, -5.1146) knots 0 0 0 0 0 0 0.014286 0.028571 0.042857 0.057143 0.071429 0.085714 0.1 0.114286 0.128571 0.142857 0.157143 0.171429 0.185714 0.2 0.214286 0.228571 0.242857 0.257143 0.271429 0.285714 0.3 0.314286 0.328571 0.342857 0.357143 0.371429 0.385714 0.4 0.414286 0.428571 0.442857 0.457143 0.471429 0.485714 0.5 0.514286 0.528571 0.542857 0.557143 0.571429 0.585714 0.6 0.614286 0.628571 0.642857 0.657143 0.671429 0.685714 0.7 0.714286 0.728571 0.742857 0.757143 0.771429 0.785714 0.8 0.814286 0.828571 0.842857 0.857143 0.871429 0.885714 0.9 0.914286 0.928571 0.942857 0.957143 1 1 1 1 1 1
  arc A19 (-3.1371, -5.1146) -> (-2.9459, -5.227) centre (0, 0) ccw
  spline S19 degree 5 poles (-2.4539, -4.7611) (-2.4547, -4.7627) (-2.4565, -4.766) (-2.4592, -4.7709) (-2.4631, -4.7772) (-2.4681, -4.785) (-2.4733, -4.7927) (-2.4787, -4.8003) (-2.4841, -4.8079) (-2.4896, -4.8155) (-2.4952, -4.823) (-2.5008, -4.8305) (-2.5065, -4.838) (-2.5123, -4.8454) (-2.5182, -4.8528) (-2.5242, -4.8601) (-2.5302, -4.8673) (-2.5364, -4.8745) (-2.5425, -4.8817) (-2.5488, -4.8889) (-2.5551, -4.896) (-2.5614, -4.9031) (-2.5678, -4.9102) (-2.5743, -4.9172) (-2.5808, -4.9242) (-2.5874, -4.9311) (-2.594, -4.9381) (-2.6007, -4.945) (-2.6074, -4.9518) (-2.6142, -4.9587) (-2.621, -4.9655) (-2.6279, -4.9723) (-2.6349, -4.979) (-2.6418, -4.9857) (-2.6489, -4.9924) (-2.6559, -4.9991) (-2.6631, -5.0057) (-2.6702, -5.0123) (-2.6774, -5.0189) (-2.6847, -5.0254) (-2.692, -5.032) (-2.6993, -5.0385) (-2.7067, -5.0449) (-2.7141, -5.0514) (-2.7216, -5.0578) (-2.7291, -5.0642) (-2.7366, -5.0705) (-2.7442, -5.0769) (-2.7518, -5.0832) (-2.7595, -5.0895) (-2.7672, -5.0957) (-2.7749, -5.102) (-2.7827, -5.1082) (-2.7905, -5.1144) (-2.7984, -5.1205) (-2.8063, -5.1266) (-2.8142, -5.1328) (-2.8222, -5.1388) (-2.8302, -5.1449) (-2.8382, -5.1509) (-2.8463, -5.1569) (-2.8544, -5.1629) (-2.8625, -5.1689) (-2.8707, -5.1748) (-2.8789, -5.1807) (-2.8872, -5.1866) (-2.8955, -5.1924) (-2.9038, -5.1983) (-2.9155, -5.2064) (-2.9256, -5.2133) (-2.934, -5.219) (-2.9408, -5.2236) (-2.9459, -5.227) knots 0 0 0 0 0 0 0.014286 0.028571 0.042857 0.057143 0.071429 0.085714 0.1 0.114286 0.128571 0.142857 0.157143 0.171429 0.185714 0.2 0.214286 0.228571 0.242857 0.257143 0.271429 0.285714 0.3 0.314286 0.328571 0.342857 0.357143 0.371429 0.385714 0.4 0.414286 0.428571 0.442857 0.457143 0.471429 0.485714 0.5 0.514286 0.528571 0.542857 0.557143 0.571429 0.585714 0.6 0.614286 0.628571 0.642857 0.657143 0.671429 0.685714 0.7 0.714286 0.728571 0.742857 0.757143 0.771429 0.785714 0.8 0.814286 0.828571 0.842857 0.857143 0.871429 0.885714 0.9 0.914286 0.928571 0.942857 0.957143 1 1 1 1 1 1
  line L19 (-2.4227, -4.7017) -> (-2.4539, -4.7611)
  arc A20 (-2.4227, -4.7017) -> (-2.1676, -4.8247) centre (0, 0) ccw
  line L20 (-2.1676, -4.8247) -> (-2.1946, -4.886)
  spline S20 degree 5 poles (-2.1946, -4.886) (-2.1953, -4.8877) (-2.1968, -4.8911) (-2.1989, -4.8963) (-2.2015, -4.9033) (-2.2045, -4.9121) (-2.2072, -4.9209) (-2.2099, -4.9299) (-2.2124, -4.9389) (-2.2149, -4.9479) (-2.2173, -4.9569) (-2.2197, -4.966) (-2.222, -4.9751) (-2.2241, -4.9843) (-2.2262, -4.9935) (-2.2282, -5.0027) (-2.2301, -5.0119) (-2.232, -5.0212) (-2.2337, -5.0305) (-2.2354, -5.0399) (-2.2371, -5.0492) (-2.2387, -5.0586) (-2.2402, -5.068) (-2.2417, -5.0775) (-2.2431, -5.0869) (-2.2444, -5.0964) (-2.2457, -5.1059) (-2.2469, -5.1154) (-2.2481, -5.125) (-2.2492, -5.1345) (-2.2503, -5.1441) (-2.2513, -5.1537) (-2.2523, -5.1634) (-2.2532, -5.173) (-2.254, -5.1827) (-2.2548, -5.1924) (-2.2556, -5.2021) (-2.2563, -5.2118) (-2.2569, -5.2215) (-2.2575, -5.2313) (-2.2581, -5.241) (-2.2586, -5.2508) (-2.2591, -5.2606) (-2.2595, -5.2704) (-2.2599, -5.2803) (-2.2602, -5.2901) (-2.2605, -5.3) (-2.2607, -5.3099) (-2.2609, -5.3198) (-2.261, -5.3297) (-2.2611, -5.3396) (-2.2612, -5.3495) (-2.2612, -5.3595) (-2.2611, -5.3694) (-2.2611, -5.3794) (-2.2609, -5.3894) (-2.2608, -5.3994) (-2.2606, -5.4094) (-2.2603, -5.4195) (-2.26, -5.4295) (-2.2597, -5.4396) (-2.2593, -5.4496) (-2.2589, -5.4597) (-2.2584, -5.4698) (-2.2579, -5.4799) (-2.2574, -5.49) (-2.2568, -5.5002) (-2.2562, -5.5103) (-2.2552, -5.5245) (-2.2544, -5.5367) (-2.2536, -5.5469) (-2.2529, -5.555) (-2.2524, -5.5612) knots 0 0 0 0 0 0 0.014286 0.028571 0.042857 0.057143 0.071429 0.085714 0.1 0.114286 0.128571 0.142857 0.157143 0.171429 0.185714 0.2 0.214286 0.228571 0.242857 0.257143 0.271429 0.285714 0.3 0.314286 0.328571 0.342857 0.357143 0.371429 0.385714 0.4 0.414286 0.428571 0.442857 0.457143 0.471429 0.485714 0.5 0.514286 0.528571 0.542857 0.557143 0.571429 0.585714 0.6 0.614286 0.628571 0.642857 0.657143 0.671429 0.685714 0.7 0.714286 0.728571 0.742857 0.757143 0.771429 0.785714 0.8 0.814286 0.828571 0.842857 0.857143 0.871429 0.885714 0.9 0.914286 0.928571 0.942857 0.957143 1 1 1 1 1 1
  arc A21 (-2.2524, -5.5612) -> (-2.0454, -5.6406) centre (0, 0) ccw
  spline S21 degree 5 poles (-1.6368, -5.1) (-1.6374, -5.1018) (-1.6385, -5.1053) (-1.6404, -5.1106) (-1.6432, -5.1175) (-1.6469, -5.126) (-1.6507, -5.1345) (-1.6548, -5.1429) (-1.6589, -5.1512) (-1.6631, -5.1596) (-1.6673, -5.1679) (-1.6716, -5.1763) (-1.676, -5.1846) (-1.6805, -5.1928) (-1.6851, -5.2011) (-1.6898, -5.2092) (-1.6946, -5.2174) (-1.6994, -5.2255) (-1.7043, -5.2336) (-1.7093, -5.2417) (-1.7144, -5.2498) (-1.7194, -5.2578) (-1.7246, -5.2658) (-1.7298, -5.2738) (-1.7351, -5.2818) (-1.7404, -5.2898) (-1.7458, -5.2977) (-1.7513, -5.3056) (-1.7568, -5.3135) (-1.7624, -5.3213) (-1.768, -5.3292) (-1.7737, -5.337) (-1.7794, -5.3448) (-1.7852, -5.3526) (-1.791, -5.3603) (-1.7969, -5.368) (-1.8028, -5.3758) (-1.8088, -5.3835) (-1.8148, -5.3911) (-1.8209, -5.3988) (-1.827, -5.4064) (-1.8332, -5.414) (-1.8394, -5.4216) (-1.8457, -5.4292) (-1.852, -5.4368) (-1.8583, -5.4443) (-1.8647, -5.4518) (-1.8711, -5.4593) (-1.8776, -5.4668) (-1.8841, -5.4743) (-1.8907, -5.4817) (-1.8973, -5.4891) (-1.904, -5.4965) (-1.9107, -5.5039) (-1.9174, -5.5113) (-1.9242, -5.5186) (-1.931, -5.5259) (-1.9378, -5.5333) (-1.9447, -5.5405) (-1.9517, -5.5478) (-1.9587, -5.5551) (-1.9657, -5.5623) (-1.9727, -5.5695) (-1.9798, -5.5767) (-1.9869, -5.5839) (-1.9941, -5.591) (-2.0013, -5.5982) (-2.0086, -5.6053) (-2.0188, -5.6152) (-2.0276, -5.6237) (-2.035, -5.6308) (-2.0409, -5.6364) (-2.0454, -5.6406) knots 0 0 0 0 0 0 0.014286 0.028571 0.042857 0.057143 0.071429 0.085714 0.1 0.114286 0.128571 0.142857 0.157143 0.171429 0.185714 0.2 0.214286 0.228571 0.242857 0.257143 0.271429 0.285714 0.3 0.314286 0.328571 0.342857 0.357143 0.371429 0.385714 0.4 0.414286 0.428571 0.442857 0.457143 0.471429 0.485714 0.5 0.514286 0.528571 0.542857 0.557143 0.571429 0.585714 0.6 0.614286 0.628571 0.642857 0.657143 0.671429 0.685714 0.7 0.714286 0.728571 0.742857 0.757143 0.771429 0.785714 0.8 0.814286 0.828571 0.842857 0.857143 0.871429 0.885714 0.9 0.914286 0.928571 0.942857 0.957143 1 1 1 1 1 1
  line L21 (-1.6158, -5.0363) -> (-1.6368, -5.1)
  arc A22 (-1.6158, -5.0363) -> (-1.3439, -5.1156) centre (0, 0) ccw
  line L22 (-1.3439, -5.1156) -> (-1.3605, -5.1806)
  spline S22 degree 5 poles (-1.3605, -5.1806) (-1.3609, -5.1824) (-1.3618, -5.186) (-1.363, -5.1915) (-1.3644, -5.1987) (-1.3659, -5.2079) (-1.3672, -5.2171) (-1.3683, -5.2264) (-1.3693, -5.2357) (-1.3703, -5.245) (-1.3712, -5.2543) (-1.372, -5.2636) (-1.3728, -5.273) (-1.3734, -5.2824) (-1.374, -5.2918) (-1.3744, -5.3012) (-1.3748, -5.3106) (-1.375, -5.3201) (-1.3753, -5.3296) (-1.3754, -5.3391) (-1.3755, -5.3486) (-1.3755, -5.3581) (-1.3755, -5.3676) (-1.3754, -5.3772) (-1.3752, -5.3867) (-1.375, -5.3963) (-1.3747, -5.4059) (-1.3743, -5.4155) (-1.3739, -5.4251) (-1.3734, -5.4347) (-1.3729, -5.4444) (-1.3723, -5.454) (-1.3717, -5.4636) (-1.371, -5.4733) (-1.3702, -5.483) (-1.3694, -5.4927) (-1.3686, -5.5024) (-1.3677, -5.5121) (-1.3667, -5.5218) (-1.3657, -5.5315) (-1.3647, -5.5412) (-1.3636, -5.551) (-1.3624, -5.5607) (-1.3612, -5.5705) (-1.3599, -5.5802) (-1.3586, -5.59) (-1.3573, -5.5998) (-1.3559, -5.6095) (-1.3544, -5.6193) (-1.3529, -5.6291) (-1.3514, -5.6389) (-1.3498, -5.6487) (-1.3482, -5.6586) (-1.3465, -5.6684) (-1.3448, -5.6782) (-1.343, -5.688) (-1.3412, -5.6979) (-1.3394, -5.7077) (-1.3375, -5.7176) (-1.3355, -5.7275) (-1.3335, -5.7373) (-1.3315, -5.7472) (-1.3294, -5.7571) (-1.3273, -5.7669) (-1.3252, -5.7768) (-1.323, -5.7867) (-1.3207, -5.7966) (-1.3184, -5.8065) (-1.3152, -5.8204) (-1.3123, -5.8323) (-1.3099, -5.8422) (-1.3079, -5.8501) (-1.3064, -5.8561) knots 0 0 0 0 0 0 0.014286 0.028571 0.042857 0.057143 0.071429 0.085714 0.1 0.114286 0.128571 0.142857 0.157143 0.171429 0.185714 0.2 0.214286 0.228571 0.242857 0.257143 0.271429 0.285714 0.3 0.314286 0.328571 0.342857 0.357143 0.371429 0.385714 0.4 0.414286 0.428571 0.442857 0.457143 0.471429 0.485714 0.5 0.514286 0.528571 0.542857 0.557143 0.571429 0.585714 0.6 0.614286 0.628571 0.642857 0.657143 0.671429 0.685714 0.7 0.714286 0.728571 0.742857 0.757143 0.771429 0.785714 0.8 0.814286 0.828571 0.842857 0.857143 0.871429 0.885714 0.9 0.914286 0.928571 0.942857 0.957143 1 1 1 1 1 1
  arc A23 (-1.3064, -5.8561) -> (-1.0891, -5.9003) centre (0, 0) ccw